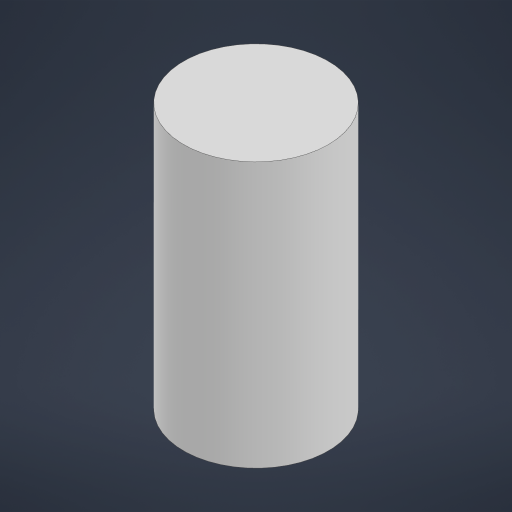
# Autodesk Inventor part: bar_holder
Saved by Autodesk Inventor 2023 (Build 270158030, 158C)
## iProperties
Created: 2022-07-16
Part Number: bar_holder
Material: Generic
Document SubType Name: Modeling
Designer: Norbert Ligas
Density: 1 g/cm^3
Appearance: Default
Author: Norbert Ligas
Autodesk Inventor part; units mm, degrees
ref_plane "YZ Plane" through (0, 0, 0) normal (1, 0, 0) x (0, 1, 0)
ref_plane "XZ Plane" through (0, 0, 0) normal (0, 1, 0) x (-1, 0, 0)
ref_plane "XY Plane" through (0, 0, 0) normal (0, 0, 1) x (1, 0, 0)
sketch "Sketch1" plane through (0, 0, 0) normal (0, 1, 0) x (-1, 0, 0)
  circle A0 centre (0, 0) radius 4
  circle A1 centre (0, 0) radius 6
  dimension "d0" = 8
  dimension "d1" = 2
  constraints: 2 centre point, 2 coincident
  measures "d0" diameter of A0
  measures "d1" radial gap between concentric circles of A1 A0
extrude "Extrusion1" add sketch "Sketch1" along normal blind 20
sketch "Sketch2" plane through (0, 20, 0) normal (0, 1, 0) x (1, 0, 0)
  circle A0 centre (0, 0) radius 4 projected
  circle A1 centre (0, 0) radius 6 projected
  circle A2 centre (0, 0) radius 6 projected
  circle A3 centre (0, 0) radius 6
  constraints: 1 centre point, 1 coincident, 1 concentric
extrude "Extrusion2" add sketch "Sketch2" along normal blind 2 contours A0 | A1
equation "\"d0\" = bar_diameter"
equation "\"d1\" = wall_thickness"
equation "\"d2\" = holder_depth"
equation "\"d4\" = wall_thickness"
equation "\"bar_diameter\" = 8"
equation "\"wall_thickness\" = 2"
equation "\"holder_depth\" = 20"
equation "\"holder_length\" = holder_depth + wall_thickness"
body "Solid1"
